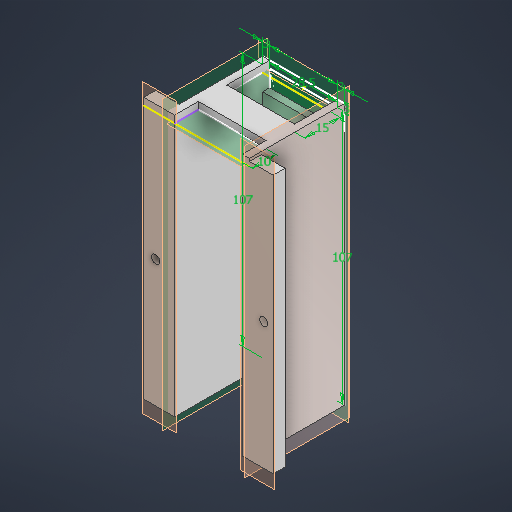
# Autodesk Inventor part: suport_batterie_2
Saved by Autodesk Inventor 2026.1 (Build 301233000, 233)
## iProperties
Created: 2026-03-10
Part Number: suport_batterie_2
Material: Generic
Document SubType Name: Modeling
Designer: fheli
Density: 1 g/cm^3
Appearance: Default
Author: fheli
Autodesk Inventor part; units mm, degrees
ref_plane "YZ Plane" through (0, 0, 0) normal (1, 0, 0) x (0, 1, 0)
ref_plane "XZ Plane" through (0, 0, 0) normal (0, 1, 0) x (-1, 0, 0)
ref_plane "XY Plane" through (0, 0, 0) normal (0, 0, 1) x (1, 0, 0)
sketch "Sketch1" plane through (0, 0, 0) normal (0, 0, 1) x (1, 0, 0)
  point P0 (0, 0)
sketch "Sketch2" plane through (0, 0, 0) normal (0, 0, 1) x (1, 0, 0)
  line L0 (-14.25, -53.5) -> (14.25, -53.5)
  line L1 (14.25, -53.5) -> (14.25, 53.5)
  line L2 (14.25, 53.5) -> (-14.25, 53.5)
  line L3 (-14.25, 53.5) -> (-14.25, -53.5)
  line L4 (-14.25, -53.5) -> (14.25, 53.5) construction
  line L5 (14.25, -53.5) -> (-14.25, 53.5) construction
  line L6 (14.25, -53.5) -> (17.25, -53.5)
  line L7 (17.25, -53.5) -> (17.25, 53.5)
  line L8 (17.25, 53.5) -> (14.25, 53.5)
  line L9 (14.25, 53.5) -> (14.25, -53.5)
  line L10 (-14.25, -53.5) -> (-17.25, -53.5)
  line L11 (-17.25, -53.5) -> (-17.25, 53.5)
  line L12 (-17.25, 53.5) -> (-14.25, 53.5)
  line L13 (-14.25, 53.5) -> (-14.25, -53.5)
  line L14 (-17.25, 53.5) -> (17.25, 53.5)
  line L15 (17.25, 53.5) -> (17.25, 56.5)
  line L16 (17.25, 56.5) -> (-17.25, 56.5)
  line L17 (-17.25, 56.5) -> (-17.25, 53.5)
  point P0 (0, 0)
  dimension "d0" = 28.5
  dimension "d1" = 107
  dimension "d2" = 3
  dimension "d3" = 3
  dimension "d4" = 107
  dimension "d5" = 3
  constraints: 36 end point, 8 parallel, 4 horizontal, 4 perpendicular, 2 midpoint, 1 point on line
  measures "d0" distance of L2.end L1.end
  measures "d1" distance of L1.end L0.end
  measures "d2" distance of L8.end L7.end
  measures "d3" distance of L11.end L12.end
  measures "d4" distance of L10.end L11.end
  measures "d5" distance of L15.end L14.end
extrude "Extrusion1" add sketch "Sketch2" along normal blind 40 contours L10 L11 L12 L3 | L1 L8 L7 L6 | L12 L17 L16 L15 L8 L2
extrude "Extrusion2" add sketch "Sketch2" along normal blind 3 contours L3 L2 L1 L0
ref_plane "Work Plane1" through (-17.25, -53.5, 0) normal (-1, 0, 0) x (0, 0, 1)
sketch "Sketch3" plane through (-17.25, -53.5, 0) normal (-1, 0, 0) x (0, 0, 1)
  line L0 (0, 110) -> (40, 110) projected
  line L1 (0, 0) -> (40, 0) projected
  line L2 (40, 110) -> (35, 110)
  line L3 (35, 110) -> (35, 0)
  line L4 (35, 0) -> (40, 0)
  line L5 (40, 0) -> (40, 110)
  point P0 (0, 53.5)
  dimension "d11" = 5
  constraints: 8 end point, 2 parallel, 1 horizontal, 1 perpendicular, 1 point on line
  measures "d11" distance of L4.end L3.end
extrude "Extrusion3" add sketch "Sketch3" along normal blind 10
ref_plane "Work Plane2" through (17.25, -53.5, 0) normal (1, 0, 0) x (0, 0, -1)
sketch "Sketch4" plane through (17.25, -53.5, 0) normal (1, 0, 0) x (0, 0, -1)
  line L0 (-40, 0) -> (-40, 110) projected
  line L1 (-40, 0) -> (-35, 0)
  line L2 (-35, 0) -> (-35, 108.8698)
  line L3 (-35, 108.8698) -> (-40, 108.8698)
  line L4 (-40, 108.8698) -> (-40, 0)
  point P0 (0, 53.5)
  dimension "d15" = 5
  constraints: 8 end point, 2 parallel, 1 horizontal, 1 perpendicular
  measures "d15" distance of L3.end L2.end
extrude "Extrusion4" add sketch "Sketch4" along normal blind 10
ref_plane "Work Plane3" through (-14.25, 53.5, 40) normal (0, -1, 0) x (1, 0, 0)
sketch "Sketch5" plane through (-14.25, 53.5, 40) normal (0, -1, 0) x (1, 0, 0)
  line L0 (0, -37) -> (28.5, -37) projected
  line L1 (28.5, -37) -> (28.5, 0) projected
  line L2 (0, -37) -> (28.5, -37)
  line L3 (28.5, -37) -> (28.5, -22)
  line L4 (28.5, -22) -> (0, -22)
  line L5 (0, -22) -> (0, -37)
  line L6 (31.5, 0) -> (-13, 0) projected
  line L7 (0, 0) -> (28.5, 0)
  line L8 (28.5, 0) -> (28.5, -10)
  line L9 (28.5, -10) -> (0, -10)
  line L10 (0, -10) -> (0, 0)
  point P0 (14.25, -40)
  dimension "d19" = 15
  dimension "d20" = 10
  constraints: 16 end point, 4 parallel, 3 point on line, 2 horizontal, 2 perpendicular
  measures "d19" distance of L3.end L2.end
  measures "d20" distance of L7.end L8.end
extrude "Extrusion5" cut sketch "Sketch5" against normal blind 10 contours L5 L4 L1 L0
extrude "Extrusion6" cut sketch "Sketch5" against normal blind 10 contours L9 L10 L6 L1
ref_plane "Work Plane4" through (0, 0, 0) normal (0, 0, -1) x (-1, 0, 0)
sketch "Sketch6" plane through (0, 0, 0) normal (0, 0, -1) x (-1, 0, 0)
  line L0 (-14.25, 53.5) -> (-14.25, 56.5) projected
  line L1 (14.25, -53.5) -> (14.25, 56.5) projected
  line L2 (-14.25, 56.5) -> (14.25, 56.5)
  line L3 (14.25, 56.5) -> (14.25, 46.5)
  line L4 (14.25, 46.5) -> (-14.25, 46.5)
  line L5 (-14.25, 46.5) -> (-14.25, 56.5)
  point P0 (0, 0)
  point P1 (14.25, 56.5)
  dimension "d26" = 10
  constraints: 8 end point, 2 parallel, 1 horizontal, 1 perpendicular, 1 point on line
  measures "d26" distance of L2.end L3.end
extrude "Extrusion7" cut sketch "Sketch6" against normal blind 10
ref_plane "Work Plane5" through (0, 0, 40) normal (0, 0, 1) x (1, 0, 0)
ref_plane "Work Plane6" through (0, 0, 40) normal (0, 0, 1) x (1, 0, 0)
sketch "Sketch7" plane through (0, 0, 40) normal (0, 0, 1) x (1, 0, 0)
  circle A0 centre (23.25, 0) radius 1.75
  point P0 (0, 0)
  dimension "d31" = 3.5
  constraints: 1 centre point
  measures "d31" diameter of A0
sketch "Sketch8" plane through (0, 0, 40) normal (0, 0, 1) x (1, 0, 0)
  circle A0 centre (-22.25, 0) radius 1.75
  point P0 (0, 0)
  dimension "d32" = 3.5
  constraints: 1 centre point
  measures "d32" diameter of A0
extrude "Extrusion8" cut sketch "Sketch8" against normal blind 10
extrude "Extrusion9" cut sketch "Sketch7" against normal blind 10
body "Solid1"
